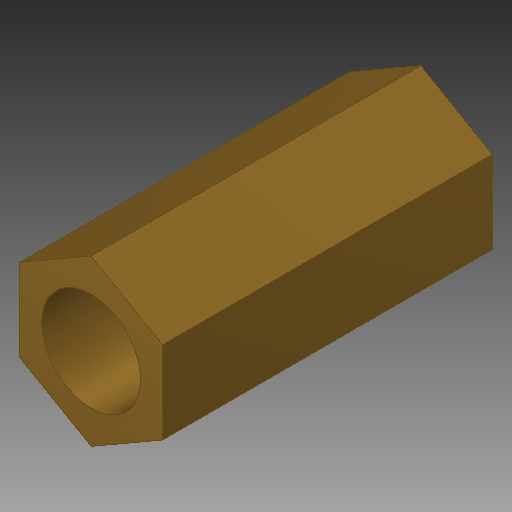
# Autodesk Inventor part: стойка для платы 10мм
Saved by Autodesk Inventor 2019 (Build 230136000, 136)
## iProperties
Created: 2018-05-25
Part Number: стойка для платы 10мм
Material: Латунь, мягкая, желтая
Document SubType Name: Modeling
Designer: olege
Density: 8.47 g/cm^3
Appearance: Латунь - сатинированная
Author: olege
Autodesk Inventor part; units mm, degrees
ref_plane "YZ Plane" through (0, 0, 0) normal (1, 0, 0) x (0, 1, 0)
ref_plane "XZ Plane" through (0, 0, 0) normal (0, 1, 0) x (-1, 0, 0)
ref_plane "XY Plane" through (0, 0, 0) normal (0, 0, 1) x (1, 0, 0)
sketch "Эскиз1" plane through (0, 0, 0) normal (0, 0, 1) x (1, 0, 0)
  circle A0 centre (0, 0) radius 1.5
  circle A1 centre (0, 0) radius 2.5 construction
  line L0 (-2.1651, 1.25) -> (0, 2.5)
  line L1 (0, 2.5) -> (2.1651, 1.25)
  line L2 (2.1651, 1.25) -> (2.1651, -1.25)
  line L3 (2.1651, -1.25) -> (0, -2.5)
  line L4 (0, -2.5) -> (-2.1651, -1.25)
  line L5 (-2.1651, -1.25) -> (-2.1651, 1.25)
  dimension "d1" = 5
  dimension "d0" = 3
  constraints: 12 end point, 3 coincident, 1 centre point, 1 vertical, 16 other
  measures "d0" diameter of A0
extrude "Выдавливание1" add sketch "Эскиз1" along normal blind 10
